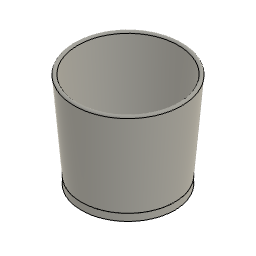
TervisHolder (Autodesk Fusion 360 design; units mm, degrees)
Autodesk Fusion 360 part; units mm, degrees
note: some values were not read from the file. Chosen so that the rebuilt part matches the saved one: which sketch regions a step uses; which face or edge a step refers to.
sketch "Sketch1" plane through (0, 0, 0) normal (0, 0, 1) x (1, 0, 0)
  circle A0 centre (0, 0) radius 39.75
  circle A1 centre (0, 0) radius 36.75
  dimension "d6" = 79.5
  dimension "d9" = 73.5
  constraint coincident A0.centre A1.centre
  constraint concentric A0 A1
  measures "d6" diameter of A0
  measures "d9" diameter of A1
ref_plane "WorkPlane1" through (0, 0, 76) normal (0, 0, 1) x (1, 0, 0)
sketch "Sketch2" plane through (0, 0, 76) normal (0, 0, 1) x (1, 0, 0)
  circle A0 centre (0, 0) radius 46.05
  circle A1 centre (0, 0) radius 43.05
  dimension "d8" = 92.1
  dimension "d10" = 86.1
  constraint coincident A0.centre A1.centre
  constraint concentric A0 A1
  measures "d8" diameter of A0
  measures "d10" diameter of A1
loft "Loft1" add profiles "Sketch1", "Sketch2" section 1 contours A0 | A1 section 2 makes body 1
loft "Loft2" cut profiles "Sketch2", "Sketch1" section 1 contours A1 section 2 contours A1 bodies 1
extrude "Extrude1" add sketch "Sketch1" against normal blind 6 separate body contours A0 | A1 makes body 2
fillet "Fillet1" radius 1.5 2 edges at (-43.05, 0, 76) (-46.05, 0, 76) on bodies 1
equation "bottomID = 70 mm"
equation "topID = 82 mm"
equation "innerHeight = 70 mm"
equation "fudge = 0.05"
equation "wall = 3 mm"
equation "d6 = bottomID + bottomID * fudge + wall * 2"
equation "d7 = innerHeight + 2 * wall"
equation "d8 = topID + topID * fudge + 2 * wall"
equation "d9 = bottomID + bottomID * fudge"
equation "d10 = topID + topID * fudge"
equation "d11 = -wall * 2"
